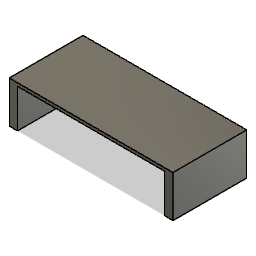
Battery_Bracket (Autodesk Fusion 360 design; units mm, degrees)
Autodesk Fusion 360 part; units mm, degrees
sketch "Sketch1" plane through (0, 0, 0) normal (0, 1, 0) x (1, 0, 0)
  line L0 (-25.4646, 4.2269) -> (74.3574, 4.2269)
  line L1 (74.3574, 4.2269) -> (74.3574, -40.7311)
  line L2 (74.3574, -40.7311) -> (-25.4646, -40.7311)
  line L3 (-25.4646, -40.7311) -> (-25.4646, 4.2269)
  dimension "d1" = 99.822
  dimension "d2" = 44.958
  constraint horizontal L0
  constraint vertical L1
  constraint horizontal L2
  constraint vertical L3
  measures "d1" distance of L0.start L0.end
  measures "d2" distance of L0.start L2.end
extrude "Extrude1" add sketch "Sketch1" along normal blind 25.4
sketch "Sketch2" plane through (0, 0, 40.7311) normal (0, 0, 1) x (1, 0, 0)
  line L0 (-25.4646, 0) -> (74.3574, 0)
  line L1 (74.3574, 0) -> (74.3574, 25.4)
  line L2 (74.3574, 25.4) -> (-25.4646, 25.4)
  line L3 (-25.4646, 25.4) -> (-25.4646, 0)
  line L4 (-20.3846, 23.495) -> (69.2774, 23.495)
  line L5 (69.2774, 23.495) -> (69.2774, 0)
  line L6 (69.2774, 0) -> (-20.3846, 0)
  line L7 (-20.3846, 0) -> (-20.3846, 23.495)
  dimension "d5" = 5.08
  dimension "d6" = 5.08
  dimension "d7" = 1.905
  constraint horizontal L4
  constraint vertical L5
  constraint horizontal L6
  constraint vertical L7
  constraint coincident L0 L5.end
  measures "d5" distance of L3 L7
  measures "d6" distance of L1 L5
  measures "d7" distance of L2 L4
extrude "Extrude2" cut sketch "Sketch2" against normal blind 66.04 contours L0 L4 L5 L6 L7
